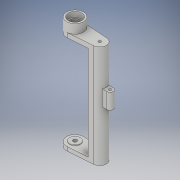
# Autodesk Inventor part: Servo-Arm-Mouth
Saved by Autodesk Inventor 2018.3 (Build 223284000, 284)
## iProperties
Created: 2018-02-17
Part Number: Servo-Arm-Mouth
Material: Generisch
Document SubType Name: Modeling
Designer: JochenAlt
Density: 1 g/cm^3
Appearance: Vorgabe
Author: JochenAlt
Autodesk Inventor part; units mm, degrees
ref_plane "YZ Plane" through (0, 0, 0) normal (1, 0, 0) x (0, 1, 0)
ref_plane "XZ Plane" through (0, 0, 0) normal (0, 1, 0) x (-1, 0, 0)
sketch "Skizze1" plane through (0, 0, 0) normal (0, 0, 1) x (1, 0, 0)
  line L0 (0, 5.6) -> (0, -5.6) construction
  line L1 (-9.12, 0) -> (26.72, 0) construction
  circle A0 centre (0, 0) radius 2
  circle A1 centre (9.5, 0) radius 1
  circle A2 centre (16, 0) radius 1
  circle A3 centre (19, 0) radius 1
  arc A4 (19.1916, -2.5929) -> (19.1916, 2.5929) centre (19, 0) ccw
  arc A5 (0.2947, 3.9891) -> (0.2947, -3.9891) centre (0, 0) ccw
  line L2 (0.2947, 3.9891) -> (19.1916, 2.5929)
  line L3 (0.2947, -3.9891) -> (19.1916, -2.5929)
  circle A6 centre (12.8, 0) radius 1
  circle A7 centre (0, 0) radius 4
  point P0 (0.5263, 3.9652)
  point P1 (0.6579, -1.8887)
  point P2 (0.6579, 1.8887)
  dimension "d0" = 9.5
  dimension "d1" = 16
  dimension "d2" = 19
  dimension "d3" = 5.2
  dimension "d4" = 2
  dimension "d5" = 4
  dimension "d6" = 8
  dimension "d17" = 12.8
  constraints: 7 centre point, 7 point on circle, 4 coincident, 4 end point, 4 point on line, 4 tangent, 3 equal radius, 3 other
  measures "d0" distance of A1.centre point (0, 0)
  measures "d1" distance of point (0, 0) A2.centre
  measures "d2" distance of A3.centre point (0, 0)
  measures "d3" diameter of A4
  measures "d4" diameter of A3
  measures "d5" diameter of A0
  measures "d6" diameter of A5
  measures "d17" distance of A6.centre point (0, 0)
extrude "Extrusion1" add sketch "Skizze1" along normal blind 1.8
extrude "Extrusion2" add sketch "Skizze1" against normal blind 2.7 contours A5 A7
sketch "Skizze6" plane through (0, 0, 0) normal (0, 0, 1) x (1, 0, 0)
  line L0 (0.2947, 3.9891) -> (19.1916, 2.5929) construction
  arc A0 (19.1916, -2.5929) -> (19.1916, 2.5929) centre (19, 0) ccw construction
  line L1 (19.1916, -2.5929) -> (0.2947, -3.9891) construction
  arc A1 (0.2947, -3.9891) -> (0.2947, 3.9891) centre (0, 0) ccw construction
  circle A2 centre (12.8, 0) radius 1 construction
  circle A3 centre (19, 0) radius 1 construction
  circle A4 centre (16, 0) radius 1 construction
  circle A5 centre (9.5, 0) radius 1 construction
  arc A6 (19.1989, -2.6927) -> (19.1989, 2.6927) centre (19, 0) ccw
  line L2 (19.1989, 2.6927) -> (0.3021, 4.0889)
  line L3 (19.3758, 5.0861) -> (0.4789, 6.4823)
  line L4 (0.4789, -6.4823) -> (19.3758, -5.0861)
  circle A7 centre (9.5, 0) radius 1 construction
  circle A8 centre (19, 0) radius 1
  line L5 (-12.62, 0) -> (30.22, 0) construction
  arc A9 (0.4789, 6.4823) -> (0.4789, -6.4823) centre (0, 0) ccw
  arc A10 (0.3021, 4.0889) -> (0.3021, -4.0889) centre (0, 0) ccw
  line L6 (0.3021, -4.0889) -> (19.1989, -2.6927)
  circle A11 centre (0, 0) radius 2 construction
  circle A12 centre (0, 0) radius 4.1
  circle A13 centre (0, 0) radius 1.25
  arc A14 (19.3758, -5.0861) -> (19.3758, 5.0861) centre (19, 0) ccw
  circle A15 centre (0, 0) radius 1.5
  dimension "d106" = 2.5
  dimension "d116" = 0.1
  dimension "d183" = 6.5
  dimension "d205" = 3
  constraints: 10 centre point, 8 coincident, 8 end point, 8 point on circle, 8 tangent, 4 concentric, 2 parallel, 1 other
  measures "d106" diameter of A13
  measures "d116" distance between parallel lines of L6 L1
  measures "d183" radius of A9
  measures "d205" diameter of A15
extrude "Extrusion11" add sketch "Skizze6" along normal blind 2 separate body contours A14 L4 A9 L3
extrude "Extrusion12" add sketch "Skizze6" along normal blind 1.5 from surface at 2 contours L6 A12 L2 A6 | A10 A12 | A14 L4 A9 L3 | A13 | A15
extrude "Extrusion16" cut sketch "Skizze6" along normal up to next contours A13
sketch "Skizze18" plane through (0, 0, 3.5) normal (0, 0, 1) x (1, 0, 0)
  circle A0 centre (0, 0) radius 5.15
  circle A1 centre (0, 0) radius 4
  circle A2 centre (0, 0) radius 6.5
  circle A3 centre (0, 0) radius 1.25 construction
  circle A4 centre (19, 0) radius 1 construction
  arc A5 (0.4789, 6.4823) -> (0.4789, -6.4823) centre (0, 0) ccw construction
  line L0 (19.3758, -5.0861) -> (0.4789, -6.4823) construction
  arc A6 (19.3758, -5.0861) -> (19.3758, 5.0861) centre (19, 0) ccw construction
  line L1 (0.4789, 6.4823) -> (19.3758, 5.0861) construction
  point P0 (-6.5, 0)
  dimension "d184" = 10.3
  dimension "d185" = 8
  constraints: 3 coincident, 2 centre point, 1 horizontal alignment, 1 point on circle, 2 other
  measures "d184" diameter of A0
  measures "d185" diameter of A1
extrude "Extrusion28" add sketch "Skizze18" along normal blind 3 contours A0 | A2
extrude "Extrusion29" add sketch "Skizze18" along normal blind 4 from surface at 3 contours A2
sketch "Skizze19" plane through (0, 0, 0) normal (0, 0, -1) x (-1, 0, 0)
  arc A0 (-19.3758, 5.0861) -> (-19.3758, -5.0861) centre (-19, 0) ccw construction
  arc A1 (-0.4789, -6.4823) -> (-0.4789, 6.4823) centre (0, 0) ccw construction
  line L0 (-0.4789, 6.4823) -> (-19.3758, 5.0861) construction
  arc A2 (-19.3758, 5.0861) -> (-19.3758, -5.0861) centre (-19, 0) ccw construction
  line L1 (-19.3758, -5.0861) -> (-0.4789, -6.4823) construction
  line L2 (-0.3021, -4.0889) -> (-19.1989, -2.6927) construction
  arc A3 (-19.1989, 2.6927) -> (-19.1989, -2.6927) centre (-19, 0) ccw construction
  line L3 (-19.1989, 2.6927) -> (-0.3021, 4.0889) construction
  arc A4 (-0.3021, -4.0889) -> (-0.3021, 4.0889) centre (0, 0) ccw construction
  arc A5 (-19.3758, 5.0861) -> (-19.3758, -5.0861) centre (-19, 0) ccw
  line L4 (-19.3758, -5.0861) -> (-15.3758, -5.3817)
  line L5 (-15.3758, -5.3817) -> (-15.1989, -2.9882)
  line L6 (-15.1989, -2.9882) -> (-19.1859, -2.6936)
  line L7 (-0.3021, -4.0889) -> (-19.1989, -2.6927) projected
  line L8 (-19.1989, 2.6927) -> (-0.3021, 4.0889) projected
  line L9 (-19.1989, 2.6927) -> (-15.1989, 2.9882)
  line L10 (-15.3758, 5.3817) -> (-19.3758, 5.0861)
  arc A6 (-19.1989, 2.6927) -> (-19.1859, -2.6936) centre (-19, 0) ccw
  line L11 (-0.4789, 6.4823) -> (-19.3758, 5.0861) projected
  line L12 (-15.1989, 2.9882) -> (-15.3758, 5.3817)
  line L13 (-19.3758, -5.0861) -> (-0.4789, -6.4823) projected
  dimension "d203" = 4
  dimension "d204" = 4
  constraints: 12 end point, 4 point on circle, 4 point on line, 3 tangent, 2 centre point, 2 coincident, 2 perpendicular
  measures "d203" horizontal distance of L4.start L4.end
  measures "d204" horizontal distance of L11.end L10.start
extrude "Extrusion30" add sketch "Skizze19" along normal blind 72.5
extrude "Extrusion31" add sketch "Skizze6" against normal blind 3 from surface at -72.5 contours L6 A12 L2 A6 | A10 A12 | A14 L4 A9 L3
extrude "Extrusion32" add sketch "Skizze6" along normal blind 0.5 from surface at -72.5 contours A10 A12
ref_plane "Arbeitsebene10" through (0, 0, -30.5) normal (0, 0, -1) x (-1, 0, 0)
sketch "Skizze20" plane through (0, 0, -30.5) normal (0, 0, -1) x (-1, 0, 0)
  arc A0 (-27, 2.5) -> (-27, -2.5) centre (-27, 0) ccw
  line L0 (-27, -2.5) -> (-19.7141, -2.5)
  line L1 (-27, 2.5) -> (-19.7141, 2.5)
  line L2 (0, -9.1) -> (0, 9.1) construction
  line L3 (-36.7, 0) -> (13.7, 0) construction
  arc A1 (-19.7141, 2.5) -> (-19.7141, -2.5) centre (-19.0084, 0) ccw
  circle A2 centre (-27, 0) radius 1.05
  arc A3 (-19.1916, 2.5929) -> (-19.1916, -2.5929) centre (-19, 0) ccw construction
  point P0 (0, 0)
  dimension "d198" = 5
  dimension "d199" = 2.1
  dimension "d200" = 27
  constraints: 5 point on circle, 4 end point, 3 centre point, 2 point on line, 2 tangent, 1 coincident, 1 horizontal, 1 parallel
  measures "d198" diameter of A0
  measures "d199" diameter of A2
  measures "d200" distance of point (0, 0) A0.centre
extrude "Extrusion33" add sketch "Skizze20" along normal mid plane 12
